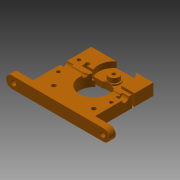
# Autodesk Inventor part: Part16
Saved by Autodesk Inventor 2015 (Build 190159000, 159)
## iProperties
Created: 2015-07-08
Part Number: Part16
Material: ABS Plastic
Document SubType Name: Modeling
Designer: eefred
Density: 1.06 g/cm^3
Appearance: Orange
Author: eefred
Autodesk Inventor part; units mm, degrees
ref_plane "YZ Plane" through (0, 0, 0) normal (1, 0, 0) x (0, 1, 0)
ref_plane "XZ Plane" through (0, 0, 0) normal (0, 1, 0) x (-1, 0, 0)
ref_plane "XY Plane" through (0, 0, 0) normal (0, 0, 1) x (1, 0, 0)
sketch "Sketch1" plane through (0, 0, 0) normal (0, 0, 1) x (1, 0, 0)
  line L0 (-24, 50) -> (24, 50)
  line L1 (24, 50) -> (24, 5)
  line L2 (-24, 5) -> (-24, 50)
  line L3 (-40, 0) -> (40, 0)
  line L4 (40, 0) -> (40, 5)
  line L5 (-40, 5) -> (-40, 0)
  line L6 (40, 5) -> (24, 5)
  line L7 (-40, 5) -> (-24, 5)
  circle A0 centre (3, 25) radius 11.3
  circle A1 centre (-20, 36.5) radius 1.35
  circle A2 centre (-20, 20.5) radius 1.35
  circle A3 centre (21, 20.5) radius 1.35
  circle A4 centre (-12.5, 9.5) radius 1.6
  circle A5 centre (18.5, 9.5) radius 1.6
  circle A6 centre (-14, 37) radius 1.5
  point P0 (0, 0)
  point P1 (0, 0)
  dimension "d0" = 50
  dimension "d1" = 48
  dimension "d2" = 80
  dimension "d3" = 16
  dimension "d4" = 5
  dimension "d5" = 22.6
  dimension "d6" = 25
  dimension "d7" = 21
  dimension "d8" = 2.7
  dimension "d9" = 16
  dimension "d10" = 4
  dimension "d11" = 4.5
  dimension "d12" = 3
  dimension "d13" = 3.2
  dimension "d14" = 31
  dimension "d15" = 11.5
  dimension "d16" = 9.5
  dimension "d17" = 3
  dimension "d18" = 10
  dimension "d19" = 12
  constraints: 16 end point, 7 centre point, 3 equal length, 3 equal radius, 3 horizontal, 3 horizontal alignment, 2 coincident, 2 perpendicular, 1 midpoint, 1 vertical alignment
  measures "d0" distance between parallel lines of L3 L0
  measures "d1" distance of L0.start L0.end
  measures "d2" distance of L3.start L3.end
  measures "d3" distance of L5.start L2.start
  measures "d4" distance of L5.start L3.start
  measures "d5" diameter of A0
  measures "d6" distance from line of L3 A0.centre
  measures "d7" distance from line of L1 A0.centre
  measures "d8" diameter of A1
  measures "d9" distance of A2.centre A1.centre
  measures "d10" distance from line of L2 A1.centre
  measures "d11" vertical distance of A0.centre A2.centre
  measures "d12" distance from line of L1 A3.centre
  measures "d13" diameter of A4
  measures "d14" distance of A5.centre A4.centre
  measures "d15" distance from line of L2 A4.centre
  measures "d16" distance from line of L3 A4.centre
  measures "d17" diameter of A6
  measures "d18" distance from line of L2 A6.centre
  measures "d19" vertical distance of A0.centre A6.centre
extrude "Extrusion1" add sketch "Sketch1" along normal blind 9
sketch "Sketch2" plane through (0, 0, 9) normal (0, 0, 1) x (1, 0, 0)
  line L0 (24, 5) -> (24, 50) projected
  line L1 (-15, 33.5) -> (24, 33.5)
  line L2 (24, 33.5) -> (24, 35.5)
  line L3 (24, 35.5) -> (-13, 35.5)
  line L4 (-13, 35.5) -> (-13, 38.5)
  line L5 (-13, 38.5) -> (-15, 38.5)
  line L6 (-15, 38.5) -> (-15, 33.5)
  line L7 (24, 50) -> (-24, 50) projected
  point P0 (0, 0)
  dimension "d22" = 14.5
  dimension "d23" = 2
  dimension "d24" = 2
  dimension "d25" = 39
  dimension "d26" = 5
  constraints: 12 end point, 2 horizontal, 2 parallel, 1 perpendicular, 1 point on line, 1 vertical
  measures "d22" distance between parallel lines of L7 L3
  measures "d23" distance between parallel lines of L1 L3
  measures "d24" distance of L4.end L5.end
  measures "d25" distance of L1.start L1.end
  measures "d26" distance of L5.end L1.start
extrude "Extrusion2" cut sketch "Sketch2" against normal through all
sketch "Sketch3" plane through (0, 0, 9) normal (0, 0, 1) x (1, 0, 0)
  circle A0 centre (3, 40.5) radius 12
  line L0 (-40, 0) -> (40, 0) projected
  line L1 (-24, 50) -> (-24, 5) projected
  point P0 (0, 0)
  dimension "d29" = 24
  dimension "d30" = 40.5
  dimension "d31" = 27
  constraints: 1 centre point
  measures "d29" diameter of A0
  measures "d30" distance from line of L0 A0.centre
  measures "d31" distance from line of L1 A0.centre
extrude "Extrusion3" cut sketch "Sketch3" against normal blind 4.5
sketch "Sketch4" plane through (0, 0, 4.5) normal (0, 0, 1) x (1, 0, 0)
  arc A0 (-4.3314, 50) -> (-7.9087, 35.5) centre (3, 40.5) ccw construction
  circle A1 centre (3, 40.5) radius 5
  point P0 (0, 0)
  dimension "d34" = 10
  constraints: 1 centre point, 1 coincident
  measures "d34" diameter of A1
extrude "Extrusion4" add sketch "Sketch4" along normal blind 1
sketch "Sketch5" plane through (3, 40.5, 5.5) normal (0, 0, 1) x (1, 0, 0)
  circle A0 centre (0, 0) radius 4
  circle A1 centre (0, 0) radius 5 construction
  point P0 (-3, -40.5)
  dimension "d37" = 8
  constraints: 1 centre point, 1 coincident
  measures "d37" diameter of A0
extrude "Extrusion5" add sketch "Sketch5" along normal blind 3.5
sketch "Sketch6" plane through (3, 40.5, 9) normal (0, 0, 1) x (1, 0, 0)
  circle A0 centre (0, 0) radius 4 construction
  arc A1 (-8.6894, -8.2761) -> (8.6894, -8.2761) centre (0, -15.5) ccw construction
  circle A2 centre (0, 0) radius 1.35
  circle A3 centre (0, -15.5) radius 11.3
  point P0 (-3, -40.5)
  dimension "d40" = 2.7
  constraints: 2 centre point, 2 coincident, 1 concentric
  measures "d40" diameter of A2
extrude "Extrusion6" cut sketch "Sketch6" against normal through all
sketch "Sketch7" plane through (-24, 5, 0) normal (-1, 0, 0) x (0, 0, 1)
  line L0 (9, 45) -> (9, 0) projected
  circle A0 centre (9, 23.5) radius 1
  line L1 (0, 45) -> (9, 45) projected
  point P0 (0, -5)
  dimension "d43" = 2
  dimension "d44" = 21.5
  constraints: 1 centre point, 1 point on line
  measures "d43" diameter of A0
  measures "d44" distance from line of L1 A0.centre
extrude "Extrusion7" cut sketch "Sketch7" against normal through all
sketch "Sketch8" plane through (-24, 5, 0) normal (-1, 0, 0) x (0, 0, 1)
  arc A0 (9, 24.5) -> (9, 22.5) centre (9, 23.5) ccw construction
  circle A1 centre (9, 23.5) radius 2.7
  point P0 (0, -5)
  dimension "d47" = 5.4
  constraints: 1 centre point, 1 coincident
  measures "d47" diameter of A1
extrude "Extrusion8" cut sketch "Sketch8" against normal blind 5
sketch "Sketch9" plane through (24, 5, 9) normal (1, 0, 0) x (0, 0, -1)
  arc A0 (0, 22.5) -> (0, 24.5) centre (0, 23.5) ccw construction
  circle A1 centre (0, 23.5) radius 2.7
  point P0 (9, -5)
  dimension "d50" = 5.4
  constraints: 1 centre point, 1 coincident
  measures "d50" diameter of A1
extrude "Extrusion9" cut sketch "Sketch9" against normal blind 5
sketch "Sketch10" plane through (0, 0, 9) normal (0, 0, 1) x (1, 0, 0)
  line L0 (-10, 29.5) -> (-6, 31.0999)
  line L1 (-6, 31.0999) -> (-6, 28.5)
  line L2 (-10, 29.5) -> (-10, 28.5)
  line L3 (-10, 28.5) -> (-6, 28.5)
  line L4 (-19, 31.2) -> (-19, 29.5) projected
  point P0 (0, 0)
  dimension "d54" = 1
  dimension "d55" = 21.8
  dimension "d56" = 9
  dimension "d57" = 4
  constraints: 8 end point, 2 vertical, 1 horizontal alignment, 1 perpendicular
  measures "d54" distance of L0.start L2.end
  measures "d55" angle of L3 L0
  measures "d56" distance between parallel lines of L4 L2
  measures "d57" distance of L2.end L1.end
revolve "Revolution1" cut sketch "Sketch10" angle 360 about axis through (-10, 28.5, 9) along (1, 0, 0)
sketch "Sketch11" plane through (-24, 50, 0) normal (0, 1, 0) x (1, 0, 0)
  circle A0 centre (43, -4.5) radius 1.6
  line L0 (48, 0) -> (48, -9) projected
  point P0 (24, 0)
  point P1 (48, -4.5)
  dimension "d59" = 3.2
  dimension "d61" = 5
  constraints: 1 centre point, 1 horizontal alignment, 1 midpoint
  measures "d59" diameter of A0
  measures "d61" distance from line of L0 A0.centre
extrude "Extrusion10" cut sketch "Sketch11" against normal up to next
sketch "Sketch12" plane through (10.4458, 33.5, 0) normal (0, 1, 0) x (1, 0, 0)
  circle A0 centre (8.5542, -4.5) radius 1.6 construction
  line L0 (-0.1144, -4.5) -> (-0.1144, -9) construction
  line L1 (13.5542, -9) -> (-0.1144, -9) construction
  line L2 (13.5542, 0) -> (13.5542, -9) construction
  line L3 (-34.4458, 0) -> (13.5542, 0) construction
  line L4 (-34.4458, 0) -> (-34.4458, -9) construction
  line L5 (-14.7772, -9) -> (-34.4458, -9) construction
  line L6 (-14.7772, -9) -> (-14.7772, -4.5) construction
  line L7 (-14.7772, -4.5) -> (-0.1144, -4.5) construction
  circle A1 centre (8.5542, -4.5) radius 1.35
  point P0 (-10.4458, 0)
  dimension "d64" = 2.7
  constraints: 1 centre point, 1 coincident
  measures "d64" diameter of A1
extrude "Extrusion11" cut sketch "Sketch12" against normal blind 13.5
fillet "Fillet1" radius 4.5 4 edges at (40, 2.5, 9) (40, 2.5, 0) (-40, 2.5, 9) (-40, 2.5, 0)
sketch "Sketch13" plane through (-35.5, 0, 0) normal (0, -1, 0) x (1, 0, 0)
  circle A0 centre (70, 4.5) radius 2.1
  circle A1 centre (1, 4.5) radius 2.1
  line L0 (71, 0) -> (0, 0) projected
  point P0 (35.5, 0)
  dimension "d68" = 4.2
  dimension "d69" = 4.5
  dimension "d70" = 69
  dimension "d71" = 34.5
  constraints: 2 centre point, 1 equal radius, 1 horizontal alignment
  measures "d68" diameter of A0
  measures "d69" distance from line of L0 A0.centre
  measures "d70" distance of A1.centre A0.centre
  measures "d71" horizontal distance of point (35.5, 0) A0.centre
extrude "Extrusion12" cut sketch "Sketch13" against normal up to next
equation "\"d71\" = 0.5 * d70"
body "Solid1"
